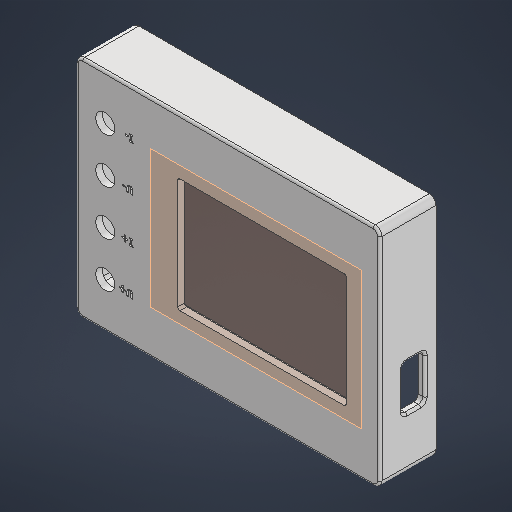
# Autodesk Inventor part: GabineteWash2
Saved by Autodesk Inventor 2026.2 (Build 302298000, 298)
## iProperties
Created: 2026-01-11
Part Number: GabineteWash2
Material: Generic
Document SubType Name: Modeling
Designer: Wellytom
Density: 1 g/cm^3
Appearance: Default
Author: Wellytom
Autodesk Inventor part; units mm, degrees
ref_plane "YZ Plane" through (0, 0, 0) normal (1, 0, 0) x (0, 1, 0)
ref_plane "XZ Plane" through (0, 0, 0) normal (0, 1, 0) x (-1, 0, 0)
ref_plane "XY Plane" through (0, 0, 0) normal (0, 0, 1) x (1, 0, 0)
ref_plane "Work Plane1" through (0, 0, 0) normal (0, 0, 1) x (1, 0, 0)
sketch "Sketch1" plane through (0, 0, 0) normal (0, 0, 1) x (1, 0, 0)
  line L0 (-99.1001, 6.92) -> (-99.1001, -63.08) projected
  line L1 (-99.1001, -63.08) -> (0.8999, -63.08) projected
  line L2 (0.8999, -63.08) -> (0.8999, 6.92) projected
  line L3 (0.8999, 6.92) -> (-99.1001, 6.92) projected
  circle A0 centre (-96.1001, -21.84) radius 0.5 projected
  circle A1 centre (-96.1001, -19.3) radius 0.5 projected
  circle A2 centre (-96.1001, -26.92) radius 0.5 projected
  circle A3 centre (-96.1001, -24.38) radius 0.5 projected
  circle A4 centre (-95.1001, 2.92) radius 1.75 projected
  circle A5 centre (-96.1001, -11.68) radius 0.5 projected
  circle A6 centre (-96.1001, -16.76) radius 0.5 projected
  circle A7 centre (-96.1001, -14.22) radius 0.5 projected
  circle A8 centre (-96.1001, -32) radius 0.5 projected
  circle A9 centre (-96.1001, -29.46) radius 0.5 projected
  circle A10 centre (-96.1001, -37.08) radius 0.5 projected
  circle A11 centre (-96.1001, -34.54) radius 0.5 projected
  circle A12 centre (-96.1001, -42.16) radius 0.5 projected
  circle A13 centre (-96.1001, -39.62) radius 0.5 projected
  circle A14 centre (-95.1001, -59.08) radius 1.75 projected
  circle A15 centre (-96.1001, -44.7) radius 0.5 projected
  circle A16 centre (-37.9001, -3.58) radius 0.4 projected
  circle A17 centre (-35.9001, -3.58) radius 0.4 projected
  circle A18 centre (-41.9001, -3.58) radius 0.4 projected
  circle A19 centre (-39.9001, -3.58) radius 0.4 projected
  circle A20 centre (-31.9001, -3.58) radius 0.4 projected
  circle A21 centre (-3.1001, 2.92) radius 1.75 projected
  circle A22 centre (-33.9001, -3.58) radius 0.4 projected
  circle A23 centre (-1.9001, -24.375) radius 0.5 projected
  circle A24 centre (-1.9001, -31.995) radius 0.5 projected
  circle A25 centre (-1.9001, -29.455) radius 0.5 projected
  circle A26 centre (-5.4501, -49) radius 0.67 projected
  circle A27 centre (-5.4501, -40.36) radius 0.67 projected
  circle A28 centre (-1.9001, -26.915) radius 0.5 projected
  circle A29 centre (-1.6501, -40.36) radius 0.67 projected
  circle A30 centre (-3.1001, -59.08) radius 1.75 projected
  circle A31 centre (-1.6501, -49) radius 0.67 projected
  line L4 (-8.98, -53.52) -> (-8.98, -2.82) projected
  line L5 (-8.98, -2.82) -> (-83.88, -2.82) projected
  line L6 (-83.88, -2.82) -> (-83.88, -53.52) projected
  line L7 (-83.88, -53.52) -> (-8.98, -53.52) projected
  line L8 (5.8999, 21.92) -> (-129.1001, 21.92)
  line L9 (-129.1001, 21.92) -> (-129.1001, -78.08)
  line L10 (-129.1001, -78.08) -> (5.8999, -78.08)
  line L11 (5.8999, -78.08) -> (5.8999, 21.92)
  point P0 (0, 0)
  point P1 (-99.1001, -28.08)
  point P2 (0.8999, -28.08)
  dimension "d0" = 135
  dimension "d1" = 100
  dimension "d2" = 50
  dimension "d3" = 5
  constraints: 8 end point, 2 midpoint, 2 parallel, 1 horizontal, 1 perpendicular
  measures "d0" distance of L9.end L10.end
  measures "d1" distance of L8.end L9.end
  measures "d2" distance from line of point (-99.1, -28.08) L10
  measures "d3" distance from line of L11 point (0.9, -28.08)
extrude "Extrusion1" add sketch "Sketch1" against normal blind 25 contours L3 L2 L1 L0 | A0 | A1 | A2 | A3 | A4 | A5 | A6 | A7 | A8 | A9 | A10 | A11 | A12 | A13 | A14 | A15 | A16 | A17 | A18 | A19 | A20 | A21 | A22 | A23 | A24 | A25 | A26 | A27 | A28 | A29 | A30 | A31 | L7 L6 L5 L4 | L11 L10 L9 L8
sketch "Sketch2" plane through (0, 0, -25) normal (0, 0, -1) x (-1, 0, 0)
  line L0 (-2.8999, 18.92) -> (126.1001, 18.92)
  line L1 (126.1001, 18.92) -> (126.1001, -75.08)
  line L2 (126.1001, -75.08) -> (-2.8999, -75.08)
  line L3 (-2.8999, -75.08) -> (-2.8999, 18.92)
  line L4 (-5.8999, 21.92) -> (-5.8999, -78.08) projected
  line L5 (-5.8999, -78.08) -> (129.1001, -78.08) projected
  line L6 (129.1001, -78.08) -> (129.1001, 21.92) projected
  line L7 (129.1001, 21.92) -> (-5.8999, 21.92) projected
  point P0 (0, 0)
  dimension "d6" = 3
  dimension "d7" = 3
  dimension "d8" = 3
  dimension "d9" = 3
  constraints: 8 end point, 2 parallel, 1 horizontal, 1 perpendicular
  measures "d6" distance between parallel lines of L4 L3
  measures "d7" distance between parallel lines of L5 L2
  measures "d8" distance between parallel lines of L6 L1
  measures "d9" distance between parallel lines of L7 L0
extrude "Extrusion2" cut sketch "Sketch2" against normal blind 22 contours L0 L1 L2 L3
sketch "Sketch3" plane through (0, 0, 0) normal (0, 0, 1) x (1, 0, 0)
  line L0 (-91.58, -55.92) -> (-91.58, -0.42) projected
  line L1 (-91.58, -55.92) -> (-6.58, -55.92) projected
  line L2 (-6.58, -55.92) -> (-6.58, -0.42) projected
  line L3 (-6.58, -0.42) -> (-91.58, -0.42) projected
  line L4 (-8.98, -53.52) -> (-8.98, -2.82) projected
  line L5 (-83.88, -53.52) -> (-8.98, -53.52) projected
  line L6 (-83.88, -2.82) -> (-83.88, -53.52) projected
  line L7 (-8.98, -2.82) -> (-83.88, -2.82) projected
  point P0 (0, 0)
extrude "Extrusion3" cut sketch "Sketch3" against normal blind 22 contours L5 L6 L7 L4
sketch "Sketch4" plane through (0, 0, 0) normal (0, 0, 1) x (1, 0, 0)
  circle A0 centre (-116.1001, -58.08) radius 4.25
  line L0 (-129.1001, -78.08) -> (5.8999, -78.08) projected
  line L1 (-129.1001, -78.08) -> (-116.1001, -78.08)
  line L2 (-116.1001, -78.08) -> (-116.1001, 21.92)
  line L3 (5.8999, 21.92) -> (-129.1001, 21.92) projected
  circle A1 centre (-116.1001, -38.08) radius 4.25
  circle A2 centre (-116.1001, -18.08) radius 4.25
  circle A3 centre (-116.1001, 1.92) radius 4.25
  point P0 (0, 0)
  point P1 (-122.6001, -78.08)
  dimension "d18" = 8.5
  dimension "d19" = 13
  dimension "d22" = 20
  dimension "d27" = 20
  constraints: 4 centre point, 4 end point, 3 point on line, 1 midpoint, 1 perpendicular, 1 vertical, 6 other
  measures "d18" diameter of A0
  measures "d19" distance of L0.start L1.end
  measures "d22" distance of A0.centre A1.centre
  measures "d27" vertical distance of point (-122.6, -78.08) A0.centre
extrude "Extrusion4" cut sketch "Sketch4" against normal blind 22
fillet "Fillet1" radius 3 8 edges at (-129.1001, -78.08, -12.5) (-129.1001, 21.92, -12.5) (5.8999, 21.92, -12.5) (5.8999, -78.08, -12.5) (2.8999, -75.08, -14) (-126.1001, -75.08, -14) (-126.1001, 18.92, -14) (2.8999, 18.92, -14)
sketch "Sketch5" plane through (0, 0, -3) normal (0, 0, -1) x (-1, 0, 0)
  circle A0 centre (3.1001, 2.92) radius 1.75 projected
  circle A1 centre (95.1001, -59.08) radius 1.75 projected
  circle A2 centre (95.1001, -59.08) radius 5
  circle A3 centre (3.1001, 2.92) radius 5
  line L0 (0, 0) -> (98, 0) projected
  line L1 (0, 0) -> (0, -56.34) projected
  line L2 (0, -56.34) -> (98, -56.34) projected
  line L3 (98, 0) -> (98, -56.34) projected
  circle A4 centre (3, -3.42) radius 1.6 projected
  circle A5 centre (96.1, -16.74) radius 0.4 projected
  circle A6 centre (96.1, -14.2) radius 0.4 projected
  circle A7 centre (96.1, -11.66) radius 0.4 projected
  circle A8 centre (1.9, -31.98) radius 0.4 projected
  circle A9 centre (1.9, -29.44) radius 0.4 projected
  circle A10 centre (1.9, -26.9) radius 0.4 projected
  circle A11 centre (1.9, -24.36) radius 0.4 projected
  circle A12 centre (95, -3.42) radius 1.6 projected
  circle A13 centre (95, -52.92) radius 1.6 projected
  circle A14 centre (3, -52.92) radius 1.6 projected
  circle A15 centre (96.1, -19.28) radius 0.4 projected
  circle A16 centre (96.1, -21.82) radius 0.4 projected
  circle A17 centre (96.1, -24.36) radius 0.4 projected
  circle A18 centre (96.1, -26.9) radius 0.4 projected
  circle A19 centre (96.1, -29.44) radius 0.4 projected
  circle A20 centre (96.1, -31.98) radius 0.4 projected
  circle A21 centre (96.1, -34.52) radius 0.4 projected
  circle A22 centre (96.1, -37.06) radius 0.4 projected
  circle A23 centre (96.1, -39.6) radius 0.4 projected
  circle A24 centre (96.1, -42.14) radius 0.4 projected
  circle A25 centre (96.1, -44.68) radius 0.4 projected
  line L4 (86.79, -57.33) -> (102.172, -57.33)
  line L5 (10.1288, 1.17) -> (-3.4706, 1.17)
  circle A26 centre (95.1001, -59.08) radius 0.5
  circle A27 centre (3.1001, 2.92) radius 0.5
  circle A28 centre (3.1001, -59.08) radius 1.75 projected
  circle A29 centre (95.1001, 2.92) radius 1.75 projected
  circle A30 centre (3.1001, -59.08) radius 5
  line L6 (-5.21, -57.33) -> (10.172, -57.33)
  circle A31 centre (3.1001, -59.08) radius 0.5
  circle A32 centre (95.1001, 2.92) radius 5
  line L7 (102.1288, 1.17) -> (88.5294, 1.17)
  circle A33 centre (95.1001, 2.92) radius 0.5
  point P0 (99.7839, -57.33)
  point P1 (90.4164, -57.33)
  point P2 (-1.5836, 1.17)
  point P3 (7.7839, 1.17)
  point P4 (-1.5836, -57.33)
  point P5 (7.7839, -57.33)
  point P6 (99.7839, 1.17)
  point P7 (90.4164, 1.17)
  dimension "d31" = 10
  dimension "d32" = 10
  dimension "d33" = 1
  dimension "d34" = 1
  dimension "d51" = 10
  dimension "d52" = 1
  dimension "d53" = 10
  dimension "d54" = 1
  constraints: 8 centre point, 8 end point, 6 coincident, 4 horizontal
  measures "d31" diameter of A2
  measures "d32" diameter of A3
  measures "d33" diameter of A26
  measures "d34" diameter of A27
  measures "d51" diameter of A30
  measures "d52" diameter of A31
  measures "d53" diameter of A32
  measures "d54" diameter of A33
extrude "Extrusion5" add sketch "Sketch5" along normal blind 5 contours A0 | L5 A3 | A29 | A32 L7 | A28 | L6 A30 | A1 | A2 L4
fillet "Fillet2" radius 2 3 edges at (-95.1001, -64.08, -3) (-3.1001, 7.92, -3) (-95.1001, 7.92, -3)
sketch "Sketch6" plane through (5.8999, -75.08, 0) normal (1, 0, 0) x (0, 0, -1)
  line L0 (16.6414, 33.54) -> (16.6414, 27.26) projected
  arc A0 (16.4914, 33.54) -> (15.3114, 34.72) centre (15.3114, 33.54) ccw projected
  line L1 (16.4914, 33.54) -> (16.4914, 27.26) projected
  arc A1 (16.6414, 33.54) -> (15.3114, 34.87) centre (15.3114, 33.54) ccw projected
  line L2 (14.8114, 34.87) -> (15.3114, 34.87) projected
  line L3 (14.8114, 34.72) -> (15.3114, 34.72) projected
  arc A2 (14.8114, 34.87) -> (13.4814, 33.54) centre (14.8114, 33.54) ccw projected
  arc A3 (14.8114, 34.72) -> (13.6314, 33.54) centre (14.8114, 33.54) ccw projected
  line L4 (13.4814, 33.54) -> (13.4814, 30.38) projected
  line L5 (13.6314, 30.38) -> (13.6314, 33.54) projected
  line L6 (13.4814, 30.37) -> (13.4814, 27.26) projected
  line L7 (13.6314, 27.26) -> (13.6314, 30.37) projected
  arc A4 (13.4814, 27.26) -> (14.8114, 25.93) centre (14.8114, 27.26) ccw projected
  arc A5 (13.6314, 27.26) -> (14.8114, 26.08) centre (14.8114, 27.26) ccw projected
  line L8 (14.8114, 25.93) -> (15.3114, 25.93) projected
  line L9 (15.3114, 26.08) -> (14.8114, 26.08) projected
  arc A6 (15.3114, 25.93) -> (16.6414, 27.26) centre (15.3114, 27.26) ccw projected
  arc A7 (15.3114, 26.08) -> (16.4914, 27.26) centre (15.3114, 27.26) ccw projected
  line L10 (15.0614, 25.93) -> (15.0614, 34.87)
  line L11 (18.0614, 40.4) -> (12.0614, 40.4)
  line L12 (10.0614, 38.4) -> (10.0614, 22.4)
  line L13 (12.0614, 20.4) -> (18.0614, 20.4)
  line L14 (20.0614, 22.4) -> (20.0614, 38.4)
  line L15 (20.0614, 40.4) -> (10.0614, 20.4) construction
  line L16 (10.0614, 40.4) -> (20.0614, 20.4) construction
  arc A8 (20.0614, 38.4) -> (18.0614, 40.4) centre (18.0614, 38.4) ccw
  arc A9 (18.0614, 20.4) -> (20.0614, 22.4) centre (18.0614, 22.4) ccw
  arc A10 (10.0614, 22.4) -> (12.0614, 20.4) centre (12.0614, 22.4) ccw
  arc A11 (12.0614, 40.4) -> (10.0614, 38.4) centre (12.0614, 38.4) ccw
  point P0 (0, 75.08)
  point P1 (15.0614, 30.4)
  dimension "d41" = 10
  dimension "d42" = 20
  dimension "d43" = 2
  constraints: 14 end point, 8 point on circle, 8 point on line, 8 tangent, 5 midpoint, 4 centre point, 3 equal radius, 2 parallel, 1 horizontal, 1 perpendicular
  measures "d41" distance of L16.end L15.end
  measures "d42" distance of L15.end L16.start
  measures "d43" radius of A8
extrude "Extrusion6" cut sketch "Sketch6" against normal blind 5 contours L0 A6 L8 L10 L9 A7 L1 A0 L3 L2 A1 | L3 A0 L1 A7 L9 L10 | A8 L14 A9 L13 A10 L12 A11 L11
fillet "Fillet3" radius 1 8 edges at (5.0212, -77.2014, 0) (5.8999, -28.08, 0) (5.0212, 21.0413, 0) (-61.6001, 21.92, 0) (-128.2214, 21.0413, 0) (-129.1001, -28.08, 0) (-128.2214, -77.2014, 0) (-61.6001, -78.08, 0)
fillet "Fillet4" radius 1 8 edges at (5.8999, -54.0942, -10.6472) (5.8999, -44.68, -10.0614) (5.8999, -35.2658, -10.6472) (5.8999, -34.68, -15.0614) (5.8999, -35.2658, -19.4756) (5.8999, -44.68, -20.0614) (5.8999, -54.0942, -19.4756) (5.8999, -54.68, -15.0614)
fillet "Fillet5" radius 1 4 edges at (-83.88, -53.52, -1.5) (-8.98, -53.52, -1.5) (-8.98, -2.82, -1.5) (-83.88, -2.82, -1.5)
sketch "Sketch7" plane through (0, 0, 0) normal (0, 0, 1) x (1, 0, 0)
  line L0 (-103.5966, -59.6361) -> (-110.1248, -59.6361) construction
  line L1 (-110.1248, -59.6361) -> (-110.1248, -56.5239) construction
  line L2 (-110.1248, -56.5239) -> (-103.5966, -56.5239) construction
  line L3 (-103.5966, -56.5239) -> (-103.5966, -59.6361) construction
  line L4 (-103.5966, -39.6361) -> (-110.1248, -39.6361) construction
  line L5 (-110.1248, -39.6361) -> (-110.1248, -36.5239) construction
  line L6 (-110.1248, -36.5239) -> (-103.5966, -36.5239) construction
  line L7 (-103.5966, -36.5239) -> (-103.5966, -39.6361) construction
  line L8 (-103.5966, -19.6361) -> (-110.1248, -19.6361) construction
  line L9 (-110.1248, -19.6361) -> (-110.1248, -16.5239) construction
  line L10 (-110.1248, -16.5239) -> (-103.5966, -16.5239) construction
  line L11 (-103.5966, -16.5239) -> (-103.5966, -19.6361) construction
  line L12 (-103.5966, 0.3639) -> (-110.1248, 0.3639) construction
  line L13 (-110.1248, 0.3639) -> (-110.1248, 3.4761) construction
  line L14 (-110.1248, 3.4761) -> (-103.5966, 3.4761) construction
  line L15 (-103.5966, 3.4761) -> (-103.5966, 0.3639) construction
  circle A0 centre (-116.1001, -58.08) radius 4.25 projected
  circle A1 centre (-116.1001, -38.08) radius 4.25 projected
  circle A2 centre (-116.1001, -18.08) radius 4.25 projected
  circle A3 centre (-116.1001, 1.92) radius 4.25 projected
  spline S0 degree 2 poles (-105.1453, -56.5239) (-104.5302, -56.5239) (-103.8683, -57.1167) (-103.8683, -57.6898) knots 0 0 0 1 2 2 2
  line L16 (-103.8683, -57.6898) -> (-103.8683, -59.6361)
  line L17 (-103.8683, -59.6361) -> (-104.634, -59.6361)
  line L18 (-104.634, -59.6361) -> (-104.634, -57.7342)
  spline S1 degree 2 poles (-104.634, -57.7342) (-104.634, -57.4156) (-104.8736, -57.1044) (-105.1453, -57.1044) knots 0 0 0 1 2 2 2
  spline S2 degree 2 poles (-105.1453, -57.1044) (-105.4095, -57.1044) (-105.6565, -57.4033) (-105.6565, -57.7342) knots 0 0 0 1 2 2 2
  line L19 (-105.6565, -57.7342) -> (-105.6565, -59.6361)
  line L20 (-105.6565, -59.6361) -> (-106.4223, -59.6361)
  line L21 (-106.4223, -59.6361) -> (-106.4223, -57.6922)
  spline S3 degree 2 poles (-106.4223, -57.6922) (-106.4223, -57.1291) (-105.7776, -56.5239) (-105.1453, -56.5239) knots 0 0 0 1 2 2 2
  line L22 (-109.7271, -57.6675) -> (-108.6798, -57.6675)
  line L23 (-108.6798, -57.6675) -> (-108.6798, -56.6277)
  line L24 (-108.6798, -56.6277) -> (-108.1389, -56.6277)
  line L25 (-108.1389, -56.6277) -> (-108.1389, -57.6675)
  line L26 (-108.1389, -57.6675) -> (-107.0916, -57.6675)
  line L27 (-107.0916, -57.6675) -> (-107.0916, -58.1961)
  line L28 (-107.0916, -58.1961) -> (-108.1389, -58.1961)
  line L29 (-108.1389, -58.1961) -> (-108.1389, -59.236)
  line L30 (-108.1389, -59.236) -> (-108.6798, -59.236)
  line L31 (-108.6798, -59.236) -> (-108.6798, -58.1961)
  line L32 (-108.6798, -58.1961) -> (-109.7271, -58.1961)
  line L33 (-109.7271, -58.1961) -> (-109.7271, -57.6675)
  line L34 (-105.4293, -36.5881) -> (-103.7892, -36.5881)
  line L35 (-103.7892, -36.5881) -> (-103.7892, -37.1192)
  line L36 (-103.7892, -37.1192) -> (-104.2264, -37.1192)
  line L37 (-104.2264, -37.1192) -> (-104.2264, -39.1051)
  line L38 (-104.2264, -39.1051) -> (-103.7892, -39.1051)
  line L39 (-103.7892, -39.1051) -> (-103.7892, -39.6361)
  line L40 (-103.7892, -39.6361) -> (-105.4293, -39.6361)
  line L41 (-105.4293, -39.6361) -> (-105.4293, -39.1051)
  line L42 (-105.4293, -39.1051) -> (-104.9921, -39.1051)
  line L43 (-104.9921, -39.1051) -> (-104.9921, -37.1192)
  line L44 (-104.9921, -37.1192) -> (-105.4293, -37.1192)
  line L45 (-105.4293, -37.1192) -> (-105.4293, -36.5881)
  line L46 (-108.6551, -37.6675) -> (-107.6079, -37.6675)
  line L47 (-107.6079, -37.6675) -> (-107.6079, -36.6277)
  line L48 (-107.6079, -36.6277) -> (-107.0669, -36.6277)
  line L49 (-107.0669, -36.6277) -> (-107.0669, -37.6675)
  line L50 (-107.0669, -37.6675) -> (-106.0196, -37.6675)
  line L51 (-106.0196, -37.6675) -> (-106.0196, -38.1961)
  line L52 (-106.0196, -38.1961) -> (-107.0669, -38.1961)
  line L53 (-107.0669, -38.1961) -> (-107.0669, -39.236)
  line L54 (-107.0669, -39.236) -> (-107.6079, -39.236)
  line L55 (-107.6079, -39.236) -> (-107.6079, -38.1961)
  line L56 (-107.6079, -38.1961) -> (-108.6551, -38.1961)
  line L57 (-108.6551, -38.1961) -> (-108.6551, -37.6675)
  spline S4 degree 2 poles (-105.1453, -16.5239) (-104.5302, -16.5239) (-103.8683, -17.1167) (-103.8683, -17.6898) knots 0 0 0 1 2 2 2
  line L58 (-103.8683, -17.6898) -> (-103.8683, -19.6361)
  line L59 (-103.8683, -19.6361) -> (-104.634, -19.6361)
  line L60 (-104.634, -19.6361) -> (-104.634, -17.7342)
  spline S5 degree 2 poles (-104.634, -17.7342) (-104.634, -17.4156) (-104.8736, -17.1044) (-105.1453, -17.1044) knots 0 0 0 1 2 2 2
  spline S6 degree 2 poles (-105.1453, -17.1044) (-105.4095, -17.1044) (-105.6565, -17.4033) (-105.6565, -17.7342) knots 0 0 0 1 2 2 2
  line L61 (-105.6565, -17.7342) -> (-105.6565, -19.6361)
  line L62 (-105.6565, -19.6361) -> (-106.4223, -19.6361)
  line L63 (-106.4223, -19.6361) -> (-106.4223, -17.6922)
  spline S7 degree 2 poles (-106.4223, -17.6922) (-106.4223, -17.1291) (-105.7776, -16.5239) (-105.1453, -16.5239) knots 0 0 0 1 2 2 2
  line L64 (-108.2748, -17.6503) -> (-106.9187, -17.6503)
  line L65 (-106.9187, -17.6503) -> (-106.9187, -18.2184)
  line L66 (-106.9187, -18.2184) -> (-108.2748, -18.2184)
  line L67 (-108.2748, -18.2184) -> (-108.2748, -17.6503)
  line L68 (-105.4293, 3.4119) -> (-103.7892, 3.4119)
  line L69 (-103.7892, 3.4119) -> (-103.7892, 2.8808)
  line L70 (-103.7892, 2.8808) -> (-104.2264, 2.8808)
  line L71 (-104.2264, 2.8808) -> (-104.2264, 0.8949)
  line L72 (-104.2264, 0.8949) -> (-103.7892, 0.8949)
  line L73 (-103.7892, 0.8949) -> (-103.7892, 0.3639)
  line L74 (-103.7892, 0.3639) -> (-105.4293, 0.3639)
  line L75 (-105.4293, 0.3639) -> (-105.4293, 0.8949)
  line L76 (-105.4293, 0.8949) -> (-104.9921, 0.8949)
  line L77 (-104.9921, 0.8949) -> (-104.9921, 2.8808)
  line L78 (-104.9921, 2.8808) -> (-105.4293, 2.8808)
  line L79 (-105.4293, 2.8808) -> (-105.4293, 3.4119)
  line L80 (-107.2028, 2.3497) -> (-105.8467, 2.3497)
  line L81 (-105.8467, 2.3497) -> (-105.8467, 1.7816)
  line L82 (-105.8467, 1.7816) -> (-107.2028, 1.7816)
  line L83 (-107.2028, 1.7816) -> (-107.2028, 2.3497)
  point P0 (0, 0)
  point P1 (-103.5966, -58.08)
  point P2 (-103.5966, -38.08)
  point P3 (-103.5966, -18.08)
  point P4 (-103.5966, 1.92)
  point P5 (-110.1248, -58.08)
  point P6 (-110.1248, -38.08)
  point P7 (-110.1248, -18.08)
  point P8 (-110.1248, 1.92)
  constraints: 8 midpoint, 4 horizontal alignment, 3 vertical alignment, 8 other
extrude "Extrusion7" cut sketch "Sketch7" against normal blind 1 contours S0 L16 L17 L18 S1 S2 L19 L20 L21 S3 | L22 L23 L24 L25 L26 L27 L28 L29 L30 L31 L32 L33 | L34 L35 L36 L37 L38 L39 L40 L41 L42 L43 L44 L45 | L46 L47 L48 L49 L50 L51 L52 L53 L54 L55 L56 L57 | S4 L58 L59 L60 S5 S6 L61 L62 L63 S7 | L64 L65 L66 L67 | L68 L69 L70 L71 L72 L73 L74 L75 L76 L77 L78 L79 | L80 L81 L82 L83
sketch "Sketch8" plane through (0, 0, -3) normal (0, 0, -1) x (-1, 0, 0)
  arc A0 (123.1001, -75.08) -> (126.1001, -72.08) centre (123.1001, -72.08) ccw projected
  circle A1 centre (123.1001, -72.08) radius 5
  circle A2 centre (123.1001, -72.08) radius 0.5
  arc A3 (126.1001, 15.92) -> (123.1001, 18.92) centre (123.1001, 15.92) ccw projected
  arc A4 (0.1001, 18.92) -> (-2.8999, 15.92) centre (0.1001, 15.92) ccw projected
  arc A5 (-2.8999, -72.08) -> (0.1001, -75.08) centre (0.1001, -72.08) ccw projected
  circle A6 centre (123.1001, 15.92) radius 5
  circle A7 centre (123.1001, 15.92) radius 0.5
  circle A8 centre (0.1001, 15.92) radius 5
  circle A9 centre (0.1001, 15.92) radius 0.5
  circle A10 centre (0.1001, -72.08) radius 5
  circle A11 centre (0.1001, -72.08) radius 0.5
  point P0 (0, 0)
  dimension "d55" = 10
  dimension "d56" = 1
  dimension "d57" = 10
  dimension "d58" = 1
  dimension "d59" = 10
  dimension "d60" = 1
  dimension "d61" = 10
  dimension "d62" = 1
  constraints: 8 centre point, 5 coincident
  measures "d55" diameter of A1
  measures "d56" diameter of A2
  measures "d57" diameter of A6
  measures "d58" diameter of A7
  measures "d59" diameter of A8
  measures "d60" diameter of A9
  measures "d61" diameter of A10
  measures "d62" diameter of A11
extrude "Extrusion8" add sketch "Sketch8" along normal blind 22
fillet "Fillet6" radius 1 12 edges at (-119.5646, -68.5445, -3) (-3.6356, -68.5445, -3) (-119.5646, 12.3844, -3) (-3.6356, 12.3844, -3) (-119.1001, 18.92, -14) (-126.1001, 11.92, -14) (-126.1001, -68.08, -14) (-119.1001, -75.08, -14) (-4.1001, -75.08, -14) (2.8999, -68.08, -14) (2.8999, 11.92, -14) (-4.1001, 18.92, -14)
body "Solid1"
